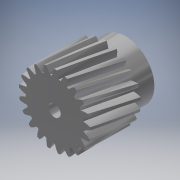
# Autodesk Inventor part: Цилиндрическое зубчатое зацепление2
Saved by Autodesk Inventor 2019 (Build 230136000, 136)
## iProperties
Created: 2019-12-26
Part Number: Цилиндрическое зубчатое зацепление2
Material: Steel
Document SubType Name: Modeling
Designer: Петров Иван
Categories: <?xml version="1.0" encoding="UTF-16"?> <MemberInstance><Categories><FamilyTemplate><FamilyTemplateParameter ValueType="xs:double" Id="1" ObjectReferenceKey="da_z" ObjectType="kUserParameterObject"/><FamilyTemplateParameter ValueType="xs:double" Id="2" ObjectReferenceKey="da_b" ObjectType="kUserParameterObject"/><FamilyTemplateParameter ValueType="xs:double" Id="3" ObjectReferenceKey="da_beta" ObjectType="kUserParameterObject"/><FamilyTemplateParameter ValueType="xs:double" Id="4" ObjectReferenceKey="da_da" ObjectType="kUserParameterObject"/><FamilyTemplateParameter ValueType="xs:double" Id="5" ObjectReferenceKey="da_aw" ObjectType="kUserParameterObject"/><FamilyTemplateParameter ValueType="xs:string" Id="6" ObjectReferenceKey="EAIAABAAAACIAQAAAAAAAIAAAAAAAAAA" ObjectType="83910656" SubObjectId="SurfaceGeometry"/></FamilyTemplate><ParamToTemplateMap><ParamToTemplate CategoryParameter="//CategoryParameter[@InternalName='046C89C9-8512-4d59-83FE-43B91F4F132A']" TemplateParameter="1"/><ParamToTemplate CategoryParameter="//CategoryParameter[@InternalName='2552DF32-E462-4b46-AEBF-C6C7768E72AC']" TemplateParameter="2"/><ParamToTemplate CategoryParameter="//CategoryParameter[@InternalName='C9EE641D-15FC-4fae-A226-E94C4372FDD7']" TemplateParameter="3"/><ParamToTemplate><ParamToTemplate CategoryParameter="//CategoryParameter[@InternalName='00B6519A-459B-49c7-AD84-2E56D39A5744']" ConstantValue="0.140671"/></ParamToTemplate><ParamToTemplate><ParamToTemplate CategoryParameter="//CategoryParameter[@InternalName='04B31F0E-C7A6-4894-AA32-9629BEFACF47']" ConstantValue="1.000000"/></ParamToTemplate><ParamToTemplate><ParamToTemplate CategoryParameter="//CategoryParameter[@InternalName='43CBEC2E-7847-49e7-A936-2F7889FCB2D9']" ConstantValue="0.250000"/></ParamToTemplate><ParamToTemplate><ParamToTemplate CategoryParameter="//CategoryParameter[@InternalName='B1EFC894-105D-4ebd-86BF-FA20ED196853']" ConstantValue="0.350000"/></ParamToTemplate><ParamToTemplate><ParamToTemplate CategoryParameter="//CategoryParameter[@InternalName='51175063-3D10-4879-93E8-6246FE8B403D']" ConstantValue="2060000000.000000"/></ParamToTemplate><ParamToTemplate><ParamToTemplate CategoryParameter="//CategoryParameter[@InternalName='A3A52E27-4454-46a9-B0BD-C932399B70AF']" ConstantValue="0.300000"/></ParamToTemplate><ParamToTemplate><ParamToTemplate CategoryParameter="//CategoryParameter[@InternalName='91B76062-C214-41d9-B1B9-14D2AB99603D']" ConstantValue="0.060000"/></ParamToTemplate><ParamToTemplate><ParamToTemplate CategoryParameter="//CategoryParameter[@InternalName='374E806E-8B8A-4dda-A9AA-1039D6500AD2']" ConstantValue="16.666667"/></ParamToTemplate><ParamToTemplate><ParamToTemplate CategoryParameter="//CategoryParameter[@InternalName='2D373A89-B862-43d6-8D0B-0CBF12AB9F6C']" ConstantValue="0.349066"/></ParamToTemplate><ParamToTemplate CategoryParameter="//CategoryParameter[@InternalName='37777632-D6A2-4fac-9D53-DB8ACD95C989']" TemplateParameter="4"/><ParamToTemplate CategoryParameter="//CategoryParameter[@InternalName='FD1017F1-B727-4f7e-9707-0F86F1FF9423']" TemplateParameter="5"/><ParamToTemplate><ParamToTemplate CategoryParameter="//CategoryParameter[@InternalName='9E1B4470-B2D3-4ff1-B813-535BB4CDF51A']" ConstantValue="3520000.000000"/></ParamToTemplate><ParamToTemplate><ParamToTemplate CategoryParameter="//CategoryParameter[@InternalName='F8452263-BFF6-458c-9FB1-07C4B99E95CD']" ConstantValue="11400000.000000"/></ParamToTemplate><ParamToTemplate><ParamToTemplate CategoryParameter="//CategoryParameter[@InternalName='3E3BB259-FD49-497f-8171-6EBC954A3479']" ConstantValue="2.000000"/></ParamToTemplate><ParamToTemplate CategoryParameter="//CategoryParameter[@InternalName='27C3BAF2-7550-4e4b-AE2C-0DB134B7D9B7']" TemplateParameter="6"/></ParamToTemplateMap><Category DisplayName="Gear" InternalName="DC85795E-93AB-48d5-8EEE-5A27447B64BD" Mnemonic="Gear"><CategoryParameter DisplayName="z" InternalName="046C89C9-8512-4d59-83FE-43B91F4F132A" Mnemonic="z"/><CategoryParameter DisplayName="b" InternalName="2552DF32-E462-4b46-AEBF-C6C7768E72AC" Mnemonic="b"/><CategoryParameter DisplayName="||b|" InternalName="C9EE641D-15FC-4fae-A226-E94C4372FDD7" Mnemonic="beta"/><CategoryParameter DisplayName="x" InternalName="00B6519A-459B-49c7-AD84-2E56D39A5744" Mnemonic="x"/><CategoryParameter DisplayName="a*" InternalName="04B31F0E-C7A6-4894-AA32-9629BEFACF47" Mnemonic="a"/><CategoryParameter DisplayName="c*" InternalName="43CBEC2E-7847-49e7-A936-2F7889FCB2D9" Mnemonic="c"/><CategoryParameter DisplayName="r|.f|*" InternalName="B1EFC894-105D-4ebd-86BF-FA20ED196853" Mnemonic="rf"/><CategoryParameter DisplayName="E" InternalName="51175063-3D10-4879-93E8-6246FE8B403D" Mnemonic="E"/><CategoryParameter DisplayName="||m|" InternalName="A3A52E27-4454-46a9-B0BD-C932399B70AF" Mnemonic="mi"/><Category DisplayName="SpurGear" InternalName="26C5A22E-A91E-4dfd-A3B3-23CCAFAE1764" Mnemonic="SpurGear"><CategoryParameter DisplayName="m" InternalName="91B76062-C214-41d9-B1B9-14D2AB99603D" Mnemonic="m"/><CategoryParameter DisplayName="P" InternalName="374E806E-8B8A-4dda-A9AA-1039D6500AD2" Mnemonic="PP"/><CategoryParameter DisplayName="||a|" InternalName="2D373A89-B862-43d6-8D0B-0CBF12AB9F6C" Mnemonic="alpha"/><CategoryParameter DisplayName="d|.a|" InternalName="37777632-D6A2-4fac-9D53-DB8ACD95C989" Mnemonic="da"/><CategoryParameter DisplayName="a|.w|" InternalName="FD1017F1-B727-4f7e-9707-0F86F1FF9423" Mnemonic="aw"/><CategoryParameter DisplayName="||s||.Flim|" InternalName="9E1B4470-B2D3-4ff1-B813-535BB4CDF51A" Mnemonic="sFlim"/><CategoryParameter DisplayName="||s||.Hlim|" InternalName="F8452263-BFF6-458c-9FB1-07C4B99E95CD" Mnemonic="sHlim"/><CategoryParameter DisplayName="тип" InternalName="3E3BB259-FD49-497f-8171-6EBC954A3479" Mnemonic="type"/><CategoryParameter DisplayName="PitchDiameter" InternalName="27C3BAF2-7550-4e4b-AE2C-0DB134B7D9B7" Mnemonic="IDS_PITCHDIAM"/></Category></Category></Categories></MemberInstance>
Density: 1 g/cm^3
Appearance: Steel
CustomPartVersion: 1
Author: Петров Иван
Autodesk Inventor part; units mm, degrees
sketch "Sketch1" plane through (0, 0, 0) normal (0, 0, 1) x (1, 0, 0)
  circle A0 centre (0, 0) radius 7.0807
  dimension "d0" = 14.1613
  constraints: 1 centre point
  measures "d0" diameter of A0
extrude "Extrusion1" add sketch "Sketch1" along normal blind 10
ref_plane "Work Plane2" through (0, 0, 5) normal (0, 0, 1) x (1, 0, 0)
sketch "Sketch2" plane through (0, 0, 0) normal (0, 0, -1) x (-1, 0, 0)
  circle A0 centre (0, 0) radius 7.0807 projected
  circle A1 centre (0, 0) radius 6.4167
  dimension "d3" = 12.8333
  constraints: 1 centre point, 1 coincident
  measures "d3" diameter of A1
surface extrude "Средний диаметр" sketch "Sketch2" against normal through all shown no curves A1
ref_plane "Work Plane8" through (0, 0, 0) normal (0.9888308, 0.1490423, 0) x (0, 0, 1)
ref_plane "Work Plane9" through (0, 0, 0) normal (1, 0, 0) x (0, 1, 0)
spur gear teeth "Цилиндрическое зубчатое зацепление" teeth 21 pitch diameter 12.7944 tip diameter 14.1613 root diameter 11.4632 face width 10 helix angle 10 hand right start plane through (0, 0, 0) normal (0, 0, -1) x (-1, 0, 0)
sketch "Эскиз3" plane through (0, 0, 10) normal (0, 0, 1) x (1, 0, 0)
  line L0 (2.8785, -0.3522) -> (2.5339, -0.4737)
  arc A0 (2.8785, -0.3522) -> (2.8942, -0.1827) centre (0, 0) ccw
  line L1 (2.5778, 0) -> (2.8942, -0.1827)
  line L2 (2.8942, 0.1827) -> (2.5778, 0)
  arc A1 (2.8942, 0.1827) -> (2.8785, 0.3522) centre (0, 0) ccw
  line L3 (2.5339, 0.4737) -> (2.8785, 0.3522)
  line L4 (2.8114, 0.7114) -> (2.5339, 0.4737)
  arc A2 (2.8114, 0.7114) -> (2.7648, 0.8752) centre (0, 0) ccw
  line L5 (2.4037, 0.9312) -> (2.7648, 0.8752)
  line L6 (2.6328, 1.2159) -> (2.4037, 0.9312)
  arc A3 (2.6328, 1.2159) -> (2.5569, 1.3683) centre (0, 0) ccw
  line L7 (2.1917, 1.357) -> (2.5569, 1.3683)
  line L8 (2.3646, 1.679) -> (2.1917, 1.357)
  arc A4 (2.3646, 1.679) -> (2.262, 1.8148) centre (0, 0) ccw
  line L9 (1.905, 1.7367) -> (2.262, 1.8148)
  line L10 (2.0158, 2.0849) -> (1.905, 1.7367)
  arc A5 (2.0158, 2.0849) -> (1.89, 2.1996) centre (0, 0) ccw
  line L11 (1.5535, 2.0571) -> (1.89, 2.1996)
  line L12 (1.5984, 2.4198) -> (1.5535, 2.0571)
  arc A6 (1.5984, 2.4198) -> (1.4536, 2.5094) centre (0, 0) ccw
  line L13 (1.149, 2.3075) -> (1.4536, 2.5094)
  line L14 (1.1265, 2.6723) -> (1.149, 2.3075)
  arc A7 (1.1265, 2.6723) -> (0.9678, 2.7338) centre (0, 0) ccw
  line L15 (0.7054, 2.4794) -> (0.9678, 2.7338)
  line L16 (0.6163, 2.8338) -> (0.7054, 2.4794)
  arc A8 (0.6163, 2.8338) -> (0.449, 2.865) centre (0, 0) ccw
  line L17 (0.2378, 2.5668) -> (0.449, 2.865)
  line L18 (0.0851, 2.8988) -> (0.2378, 2.5668)
  arc A9 (0.0851, 2.8988) -> (-0.0851, 2.8988) centre (0, 0) ccw
  line L19 (-0.2378, 2.5668) -> (-0.0851, 2.8988)
  line L20 (-0.449, 2.865) -> (-0.2378, 2.5668)
  arc A10 (-0.449, 2.865) -> (-0.6163, 2.8338) centre (0, 0) ccw
  line L21 (-0.7054, 2.4794) -> (-0.6163, 2.8338)
  line L22 (-0.9678, 2.7338) -> (-0.7054, 2.4794)
  arc A11 (-0.9678, 2.7338) -> (-1.1265, 2.6723) centre (0, 0) ccw
  line L23 (-1.149, 2.3075) -> (-1.1265, 2.6723)
  line L24 (-1.4536, 2.5094) -> (-1.149, 2.3075)
  arc A12 (-1.4536, 2.5094) -> (-1.5984, 2.4198) centre (0, 0) ccw
  line L25 (-1.5535, 2.0571) -> (-1.5984, 2.4198)
  line L26 (-1.89, 2.1996) -> (-1.5535, 2.0571)
  arc A13 (-1.89, 2.1996) -> (-2.0158, 2.0849) centre (0, 0) ccw
  line L27 (-1.905, 1.7367) -> (-2.0158, 2.0849)
  line L28 (-2.262, 1.8148) -> (-1.905, 1.7367)
  arc A14 (-2.262, 1.8148) -> (-2.3646, 1.679) centre (0, 0) ccw
  line L29 (-2.1917, 1.357) -> (-2.3646, 1.679)
  line L30 (-2.5569, 1.3683) -> (-2.1917, 1.357)
  arc A15 (-2.5569, 1.3683) -> (-2.6328, 1.2159) centre (0, 0) ccw
  line L31 (-2.4037, 0.9312) -> (-2.6328, 1.2159)
  line L32 (-2.7648, 0.8752) -> (-2.4037, 0.9312)
  arc A16 (-2.7648, 0.8752) -> (-2.8114, 0.7114) centre (0, 0) ccw
  line L33 (-2.5339, 0.4737) -> (-2.8114, 0.7114)
  line L34 (-2.8785, 0.3522) -> (-2.5339, 0.4737)
  arc A17 (-2.8785, 0.3522) -> (-2.8942, 0.1827) centre (0, 0) ccw
  line L35 (-2.5778, 0) -> (-2.8942, 0.1827)
  line L36 (-2.8942, -0.1827) -> (-2.5778, 0)
  arc A18 (-2.8942, -0.1827) -> (-2.8785, -0.3522) centre (0, 0) ccw
  line L37 (-2.5339, -0.4737) -> (-2.8785, -0.3522)
  line L38 (-2.8114, -0.7114) -> (-2.5339, -0.4737)
  arc A19 (-2.8114, -0.7114) -> (-2.7648, -0.8752) centre (0, 0) ccw
  line L39 (-2.4037, -0.9312) -> (-2.7648, -0.8752)
  line L40 (-2.6328, -1.2159) -> (-2.4037, -0.9312)
  arc A20 (-2.6328, -1.2159) -> (-2.5569, -1.3683) centre (0, 0) ccw
  line L41 (-2.1917, -1.357) -> (-2.5569, -1.3683)
  line L42 (-2.3646, -1.679) -> (-2.1917, -1.357)
  arc A21 (-2.3646, -1.679) -> (-2.262, -1.8148) centre (0, 0) ccw
  line L43 (-1.905, -1.7367) -> (-2.262, -1.8148)
  line L44 (-2.0158, -2.0849) -> (-1.905, -1.7367)
  arc A22 (-2.0158, -2.0849) -> (-1.89, -2.1996) centre (0, 0) ccw
  line L45 (-1.5535, -2.0571) -> (-1.89, -2.1996)
  line L46 (-1.5984, -2.4198) -> (-1.5535, -2.0571)
  arc A23 (-1.5984, -2.4198) -> (-1.4536, -2.5094) centre (0, 0) ccw
  line L47 (-1.149, -2.3075) -> (-1.4536, -2.5094)
  line L48 (-1.1265, -2.6723) -> (-1.149, -2.3075)
  arc A24 (-1.1265, -2.6723) -> (-0.9678, -2.7338) centre (0, 0) ccw
  line L49 (-0.7054, -2.4794) -> (-0.9678, -2.7338)
  line L50 (-0.6163, -2.8338) -> (-0.7054, -2.4794)
  arc A25 (-0.6163, -2.8338) -> (-0.449, -2.865) centre (0, 0) ccw
  line L51 (-0.2378, -2.5668) -> (-0.449, -2.865)
  line L52 (-0.0851, -2.8988) -> (-0.2378, -2.5668)
  arc A26 (-0.0851, -2.8988) -> (0.0851, -2.8988) centre (0, 0) ccw
  line L53 (0.2378, -2.5668) -> (0.0851, -2.8988)
  line L54 (0.449, -2.865) -> (0.2378, -2.5668)
  arc A27 (0.449, -2.865) -> (0.6163, -2.8338) centre (0, 0) ccw
  line L55 (0.7054, -2.4794) -> (0.6163, -2.8338)
  line L56 (0.9678, -2.7338) -> (0.7054, -2.4794)
  arc A28 (0.9678, -2.7338) -> (1.1265, -2.6723) centre (0, 0) ccw
  line L57 (1.149, -2.3075) -> (1.1265, -2.6723)
  line L58 (1.4536, -2.5094) -> (1.149, -2.3075)
  arc A29 (1.4536, -2.5094) -> (1.5984, -2.4198) centre (0, 0) ccw
  line L59 (1.5535, -2.0571) -> (1.5984, -2.4198)
  line L60 (1.89, -2.1996) -> (1.5535, -2.0571)
  arc A30 (1.89, -2.1996) -> (2.0158, -2.0849) centre (0, 0) ccw
  line L61 (1.905, -1.7367) -> (2.0158, -2.0849)
  line L62 (2.262, -1.8148) -> (1.905, -1.7367)
  arc A31 (2.262, -1.8148) -> (2.3646, -1.679) centre (0, 0) ccw
  line L63 (2.1917, -1.357) -> (2.3646, -1.679)
  line L64 (2.5569, -1.3683) -> (2.1917, -1.357)
  arc A32 (2.5569, -1.3683) -> (2.6328, -1.2159) centre (0, 0) ccw
  line L65 (2.4037, -0.9312) -> (2.6328, -1.2159)
  line L66 (2.7648, -0.8752) -> (2.4037, -0.9312)
  arc A33 (2.7648, -0.8752) -> (2.8114, -0.7114) centre (0, 0) ccw
  line L67 (2.5339, -0.4737) -> (2.8114, -0.7114)
  circle A34 centre (0, 0) radius 2.4
  circle A35 centre (0, 0) radius 2.4
  circle A36 centre (0, 0) radius 1.25
  point P0 (-10.35, -10)
  constraints: 136 end point, 68 point on circle, 37 centre point
extrude "Выдавливание2" cut sketch "Эскиз3" against normal through all contours L0 L67 A33 L66 L65 A32 L64 L63 A31 L62 L61 A30 L60 L59 A29 L58 L57 A28 L56 L55 A27 L54 L53 A26 L52 L51 A25 L50 L49 A24 L48 L47 A23 L46 L45 A22 L44 L43 A21 L42 L41 A20 L40 L39 A19 L38 L37 A18 L36 L35 A17 L34 L33 A16 L32 L31 A15 L30 L29 A14 L28 L27 A13 L26 L25 A12 L24 L23 A11 L22 L21 A10 L20 L19 A9 L18 L17 A8 L16 L15 A7 L14 L13 A6 L12 L11 A5 L10 L9 A4 L8 L7 A3 L6 L5 A2 L4 L3 A1 L2 L1 A0 | A34 | A36
sketch "Эскиз7" plane through (0, 0, 0) normal (0, 0, -1) x (-1, 0, 0)
  circle A0 centre (0, 0) radius 5.7168
  arc A1 (-2.8942, -0.1827) -> (-2.8785, -0.3522) centre (0, 0) ccw projected
  line L0 (-2.8942, -0.1827) -> (-2.5778, 0) projected
  line L1 (-2.5778, 0) -> (-2.8942, 0.1827) projected
  arc A2 (-2.8785, 0.3522) -> (-2.8942, 0.1827) centre (0, 0) ccw projected
  line L2 (-2.8785, 0.3522) -> (-2.5339, 0.4737) projected
  line L3 (-2.5339, 0.4737) -> (-2.8114, 0.7114) projected
  arc A3 (-2.7648, 0.8752) -> (-2.8114, 0.7114) centre (0, 0) ccw projected
  line L4 (-2.7648, 0.8752) -> (-2.4037, 0.9312) projected
  line L5 (-2.4037, 0.9312) -> (-2.6328, 1.2159) projected
  arc A4 (-2.5569, 1.3683) -> (-2.6328, 1.2159) centre (0, 0) ccw projected
  line L6 (-2.5569, 1.3683) -> (-2.1917, 1.357) projected
  line L7 (-2.1917, 1.357) -> (-2.3646, 1.679) projected
  arc A5 (-2.262, 1.8148) -> (-2.3646, 1.679) centre (0, 0) ccw projected
  line L8 (-2.262, 1.8148) -> (-1.905, 1.7367) projected
  line L9 (-1.905, 1.7367) -> (-2.0158, 2.0849) projected
  arc A6 (-1.89, 2.1996) -> (-2.0158, 2.0849) centre (0, 0) ccw projected
  line L10 (-1.89, 2.1996) -> (-1.5535, 2.0571) projected
  line L11 (-1.5535, 2.0571) -> (-1.5984, 2.4198) projected
  arc A7 (-1.4536, 2.5094) -> (-1.5984, 2.4198) centre (0, 0) ccw projected
  line L12 (-1.4536, 2.5094) -> (-1.149, 2.3075) projected
  line L13 (-1.149, 2.3075) -> (-1.1265, 2.6723) projected
  arc A8 (-0.9678, 2.7338) -> (-1.1265, 2.6723) centre (0, 0) ccw projected
  line L14 (-0.9678, 2.7338) -> (-0.7054, 2.4794) projected
  line L15 (-0.7054, 2.4794) -> (-0.6163, 2.8338) projected
  arc A9 (-0.449, 2.865) -> (-0.6163, 2.8338) centre (0, 0) ccw projected
  line L16 (-0.449, 2.865) -> (-0.2378, 2.5668) projected
  line L17 (-0.2378, 2.5668) -> (-0.0851, 2.8988) projected
  arc A10 (0.0851, 2.8988) -> (-0.0851, 2.8988) centre (0, 0) ccw projected
  line L18 (0.0851, 2.8988) -> (0.2378, 2.5668) projected
  line L19 (0.2378, 2.5668) -> (0.449, 2.865) projected
  arc A11 (0.6163, 2.8338) -> (0.449, 2.865) centre (0, 0) ccw projected
  line L20 (0.6163, 2.8338) -> (0.7054, 2.4794) projected
  line L21 (0.7054, 2.4794) -> (0.9678, 2.7338) projected
  arc A12 (1.1265, 2.6723) -> (0.9678, 2.7338) centre (0, 0) ccw projected
  line L22 (1.1265, 2.6723) -> (1.149, 2.3075) projected
  line L23 (1.149, 2.3075) -> (1.4536, 2.5094) projected
  arc A13 (1.5984, 2.4198) -> (1.4536, 2.5094) centre (0, 0) ccw projected
  line L24 (1.5984, 2.4198) -> (1.5535, 2.0571) projected
  line L25 (1.5535, 2.0571) -> (1.89, 2.1996) projected
  arc A14 (2.0158, 2.0849) -> (1.89, 2.1996) centre (0, 0) ccw projected
  line L26 (2.0158, 2.0849) -> (1.905, 1.7367) projected
  line L27 (1.905, 1.7367) -> (2.262, 1.8148) projected
  arc A15 (2.3646, 1.679) -> (2.262, 1.8148) centre (0, 0) ccw projected
  line L28 (2.3646, 1.679) -> (2.1917, 1.357) projected
  line L29 (2.1917, 1.357) -> (2.5569, 1.3683) projected
  arc A16 (2.6328, 1.2159) -> (2.5569, 1.3683) centre (0, 0) ccw projected
  line L30 (2.6328, 1.2159) -> (2.4037, 0.9312) projected
  line L31 (2.4037, 0.9312) -> (2.7648, 0.8752) projected
  arc A17 (2.8114, 0.7114) -> (2.7648, 0.8752) centre (0, 0) ccw projected
  line L32 (2.8114, 0.7114) -> (2.5339, 0.4737) projected
  line L33 (2.5339, 0.4737) -> (2.8785, 0.3522) projected
  arc A18 (2.8942, 0.1827) -> (2.8785, 0.3522) centre (0, 0) ccw projected
  line L34 (2.8942, 0.1827) -> (2.5778, 0) projected
  line L35 (2.5778, 0) -> (2.8942, -0.1827) projected
  arc A19 (2.8785, -0.3522) -> (2.8942, -0.1827) centre (0, 0) ccw projected
  line L36 (2.8785, -0.3522) -> (2.5339, -0.4737) projected
  line L37 (2.5339, -0.4737) -> (2.8114, -0.7114) projected
  arc A20 (2.7648, -0.8752) -> (2.8114, -0.7114) centre (0, 0) ccw projected
  line L38 (2.7648, -0.8752) -> (2.4037, -0.9312) projected
  line L39 (2.4037, -0.9312) -> (2.6328, -1.2159) projected
  arc A21 (2.5569, -1.3683) -> (2.6328, -1.2159) centre (0, 0) ccw projected
  line L40 (2.5569, -1.3683) -> (2.1917, -1.357) projected
  line L41 (2.1917, -1.357) -> (2.3646, -1.679) projected
  arc A22 (2.262, -1.8148) -> (2.3646, -1.679) centre (0, 0) ccw projected
  line L42 (2.262, -1.8148) -> (1.905, -1.7367) projected
  line L43 (1.905, -1.7367) -> (2.0158, -2.0849) projected
  arc A23 (1.89, -2.1996) -> (2.0158, -2.0849) centre (0, 0) ccw projected
  line L44 (1.89, -2.1996) -> (1.5535, -2.0571) projected
  line L45 (1.5535, -2.0571) -> (1.5984, -2.4198) projected
  arc A24 (1.4536, -2.5094) -> (1.5984, -2.4198) centre (0, 0) ccw projected
  line L46 (1.4536, -2.5094) -> (1.149, -2.3075) projected
  line L47 (1.149, -2.3075) -> (1.1265, -2.6723) projected
  arc A25 (0.9678, -2.7338) -> (1.1265, -2.6723) centre (0, 0) ccw projected
  line L48 (0.9678, -2.7338) -> (0.7054, -2.4794) projected
  line L49 (0.7054, -2.4794) -> (0.6163, -2.8338) projected
  arc A26 (0.449, -2.865) -> (0.6163, -2.8338) centre (0, 0) ccw projected
  line L50 (0.449, -2.865) -> (0.2378, -2.5668) projected
  line L51 (0.2378, -2.5668) -> (0.0851, -2.8988) projected
  arc A27 (-0.0851, -2.8988) -> (0.0851, -2.8988) centre (0, 0) ccw projected
  line L52 (-0.0851, -2.8988) -> (-0.2378, -2.5668) projected
  line L53 (-0.2378, -2.5668) -> (-0.449, -2.865) projected
  arc A28 (-0.6163, -2.8338) -> (-0.449, -2.865) centre (0, 0) ccw projected
  line L54 (-0.6163, -2.8338) -> (-0.7054, -2.4794) projected
  line L55 (-0.7054, -2.4794) -> (-0.9678, -2.7338) projected
  arc A29 (-1.1265, -2.6723) -> (-0.9678, -2.7338) centre (0, 0) ccw projected
  line L56 (-1.1265, -2.6723) -> (-1.149, -2.3075) projected
  line L57 (-1.149, -2.3075) -> (-1.4536, -2.5094) projected
  arc A30 (-1.5984, -2.4198) -> (-1.4536, -2.5094) centre (0, 0) ccw projected
  line L58 (-1.5984, -2.4198) -> (-1.5535, -2.0571) projected
  line L59 (-1.5535, -2.0571) -> (-1.89, -2.1996) projected
  arc A31 (-2.0158, -2.0849) -> (-1.89, -2.1996) centre (0, 0) ccw projected
  line L60 (-2.0158, -2.0849) -> (-1.905, -1.7367) projected
  line L61 (-1.905, -1.7367) -> (-2.262, -1.8148) projected
  arc A32 (-2.3646, -1.679) -> (-2.262, -1.8148) centre (0, 0) ccw projected
  line L62 (-2.3646, -1.679) -> (-2.1917, -1.357) projected
  line L63 (-2.1917, -1.357) -> (-2.5569, -1.3683) projected
  arc A33 (-2.6328, -1.2159) -> (-2.5569, -1.3683) centre (0, 0) ccw projected
  line L64 (-2.6328, -1.2159) -> (-2.4037, -0.9312) projected
  line L65 (-2.4037, -0.9312) -> (-2.7648, -0.8752) projected
  arc A34 (-2.8114, -0.7114) -> (-2.7648, -0.8752) centre (0, 0) ccw projected
  line L66 (-2.8114, -0.7114) -> (-2.5339, -0.4737) projected
  line L67 (-2.5339, -0.4737) -> (-2.8785, -0.3522) projected
  arc A35 (2.3386, 6.6833) -> (1.8326, 6.8394) centre (0, 0) ccw projected
  arc A36 (0.2648, 7.0757) -> (-0.2648, 7.0757) centre (0, 0) ccw projected
  arc A37 (-1.8326, 6.8394) -> (-2.3386, 6.6833) centre (0, 0) ccw projected
  arc A38 (-3.7671, 5.9954) -> (-4.2046, 5.6971) centre (0, 0) ccw projected
  arc A39 (-5.3669, 4.6186) -> (-5.6971, 4.2046) centre (0, 0) ccw projected
  arc A40 (-6.4899, 2.8315) -> (-6.6833, 2.3386) centre (0, 0) ccw projected
  arc A41 (-7.0361, 0.7928) -> (-7.0757, 0.2648) centre (0, 0) ccw projected
  arc A42 (-6.9572, -1.3164) -> (-6.8394, -1.8326) centre (0, 0) ccw projected
  arc A43 (-6.2601, -3.3086) -> (-5.9954, -3.7671) centre (0, 0) ccw projected
  arc A44 (-5.0068, -5.0068) -> (-4.6186, -5.3669) centre (0, 0) ccw projected
  arc A45 (-3.3086, -6.2601) -> (-2.8315, -6.4899) centre (0, 0) ccw projected
  arc A46 (-1.3164, -6.9572) -> (-0.7928, -7.0361) centre (0, 0) ccw projected
  arc A47 (0.7928, -7.0361) -> (1.3164, -6.9572) centre (0, 0) ccw projected
  arc A48 (2.8315, -6.4899) -> (3.3086, -6.2601) centre (0, 0) ccw projected
  arc A49 (4.6186, -5.3669) -> (5.0068, -5.0068) centre (0, 0) ccw projected
  arc A50 (5.9954, -3.7671) -> (6.2601, -3.3086) centre (0, 0) ccw projected
  arc A51 (6.8394, -1.8326) -> (6.9572, -1.3164) centre (0, 0) ccw projected
  arc A52 (7.0757, 0.2648) -> (7.0361, 0.7928) centre (0, 0) ccw projected
  arc A53 (6.6833, 2.3386) -> (6.4899, 2.8315) centre (0, 0) ccw projected
  arc A54 (5.6971, 4.2046) -> (5.3669, 4.6186) centre (0, 0) ccw projected
  arc A55 (4.2046, 5.6971) -> (3.7671, 5.9954) centre (0, 0) ccw projected
  constraints: 1 centre point, 1 coincident, 1 horizontal alignment, 62 other
extrude "Выдавливание4" add sketch "Эскиз7" along normal blind 4
sketch "Эскиз8" plane through (0, 0, 10) normal (0, 0, 1) x (1, 0, 0)
  line L0 (1.5984, 2.4198) -> (1.5535, 2.0571) projected
  circle A0 centre (0, 0) radius 2.9
  circle A1 centre (0, 0) radius 1.2
  dimension "d56" = 2.4
  constraints: 2 coincident, 1 centre point, 3 other
  measures "d56" diameter of A1
extrude "Выдавливание5" add sketch "Эскиз8" against normal blind 2
equation "\"d0\" = da_da"
equation "\"d1\" = da_b"
equation "\"d3\" = da_dw"
equation "\"d16\" = da_aw"
equation "\"d43\" = da_aw"
equation "\"d46\" = da_aw"
equation "\"da_da\" = 14.161338"
equation "\"da_b\" = 10"
equation "\"da_dw\" = 12.833333"
equation "\"da_aw\" = 27.5"
body "Solid1"
body "Srf1"
